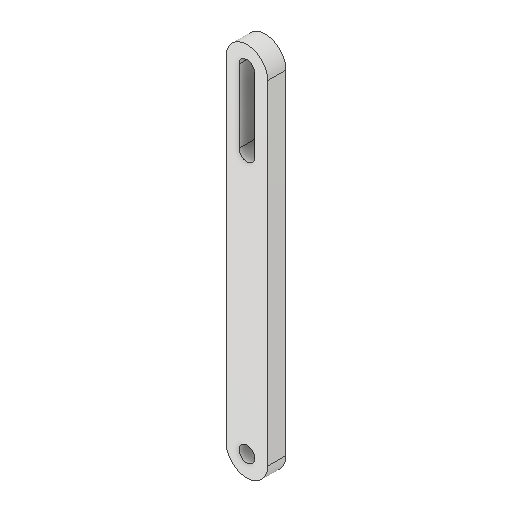
# Autodesk Inventor part: 3DP_PLA_Part_Detector_Mounting_Bracket
Saved by Autodesk Inventor 2026.1 (Build 301233000, 233)
## iProperties
Created: 2018-06-16
Part Number: 3DP_PLA_Part_Detector_Mounting_Bracket
Material: ABS Plastic
Document SubType Name: Modeling
Designer: Andrzej
Density: 1.06 g/cm^3
Appearance: Smooth - White
Author: Andrzej
Autodesk Inventor part; units mm, degrees
ref_plane "YZ Plane" through (0, 0, 0) normal (1, 0, 0) x (0, 1, 0)
ref_plane "XZ Plane" through (0, 0, 0) normal (0, 1, 0) x (-1, 0, 0)
ref_plane "XY Plane" through (0, 0, 0) normal (0, 0, 1) x (1, 0, 0)
sketch "Sketch1" plane through (0, 0, 0) normal (0, 0, 1) x (1, 0, 0)
  line L0 (0, 32) -> (0, -32) construction
  line L1 (-4, 32) -> (-4, -32)
  line L2 (4, -32) -> (4, 32)
  arc A0 (4, 32) -> (-4, 32) centre (0, 32) ccw
  arc A1 (-4, -32) -> (4, -32) centre (0, -32) ccw
  circle A2 centre (0, -32) radius 1.5
  line L3 (0, 18) -> (0, 32) construction
  line L4 (1.5, 18) -> (1.5, 32)
  line L5 (-1.5, 32) -> (-1.5, 18)
  arc A3 (-1.5, 18) -> (1.5, 18) centre (0, 18) ccw
  arc A4 (1.5, 32) -> (-1.5, 32) centre (0, 32) ccw
  point P0 (0, 0)
  point P1 (0, 25)
  dimension "d0" = 32
  dimension "d1" = 8
  dimension "d2" = 3
  dimension "d3" = 7
  dimension "d4" = 3
  dimension "d5" = 7
  constraints: 16 end point, 8 point on circle, 8 tangent, 5 centre point, 2 midpoint, 2 parallel, 2 point on line, 1 coincident, 1 vertical
  measures "d0" distance of point (0, 0) L0.end
  measures "d1" diameter of A1
  measures "d2" diameter of A2
  measures "d3" distance of point (0, 25) L3.end
  measures "d4" diameter of A4
  measures "d5" distance of L0.start point (0, 25)
extrude "Extrusion1" add sketch "Sketch1" along normal blind 3.5
body "Solid1"
